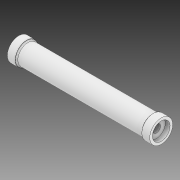
# Autodesk Inventor part: 12111_Proximal Roller_V1
Saved by Autodesk Inventor 2020 (Build 240168000, 168)
## iProperties
Created: 2019-09-30
Part Number: 12111_Proximal Roller_V1
Material: ABS Plastic
Document SubType Name: Modeling
Designer: MPI
Density: 1.06 g/cm^3
Appearance: Smooth - White
Author: MPI
Autodesk Inventor part; units mm, degrees
ref_plane "YZ Plane" through (0, 0, 0) normal (1, 0, 0) x (0, 1, 0)
ref_plane "XZ Plane" through (0, 0, 0) normal (0, 1, 0) x (-1, 0, 0)
sketch "Sketch5" plane through (0, 0, 0) normal (0, 0, 1) x (1, 0, 0)
  line L0 (71.5, 5) -> (71.5, 11.15)
  line L1 (71.5, 11.15) -> (77.5, 11.15)
  line L2 (77.5, 11.15) -> (77.5, 14.5)
  line L3 (77.5, 14.5) -> (67.5, 14.5)
  line L4 (67.5, 14.5) -> (67.5, 14.2)
  line L5 (66, 12.7) -> (-12.5, 12.7)
  line L6 (71.5, 5) -> (-12.5, 5)
  line L7 (-12.5, 5) -> (-12.5, 12.7)
  line L8 (0, 0) -> (106.4906, 0) construction
  line L9 (67.5, 14.2) -> (67.5, 14.2)
  arc A0 (66, 12.7) -> (67.5, 14.2) centre (66, 14.2) ccw
  line L10 (35.25, 16.2) -> (60.7131, 16.2)
  point P0 (67.5, 12.7)
  point P1 (67.5, 14.5)
  point P2 (67.5, 14.2)
  dimension "d12" = 5
  dimension "d14" = 6
  dimension "d16" = 11.15
  dimension "d17" = 14.5
  dimension "d19" = 10
  dimension "d27" = 80
  dimension "d28" = 1.5
  dimension "d29" = 12.7
  dimension "d30" = 3.5
  constraints: 22 end point, 4 horizontal, 4 perpendicular, 2 point on circle, 2 point on line, 2 tangent, 2 vertical, 1 centre point
  measures "d12" distance from line of L8.start L6
  measures "d14" distance between parallel lines of L2 L0
  measures "d16" distance from line of L1 L8.start
  measures "d17" distance from line of L3 L8.start
  measures "d19" distance of L2.end L3.end
  measures "d27" distance of point (67.5, 12.7) L5.end
  measures "d28" radius of A0
  measures "d29" distance from line of L8.start L5
  measures "d30" distance between parallel lines of L5 L10
revolve "Revolution1" add sketch "Sketch5" angle 360 about axis through (0, 0, 0) along (1, 0, 0)
ref_plane "Work Plane1" through (-12.5, 0, 0) normal (-1, 0, 0) x (0, 0, 1)
mirror "Mirror1" about plane through (-12.5, 0, 0) normal (-1, 0, 0) of "Revolution1"
body "Solid2"
